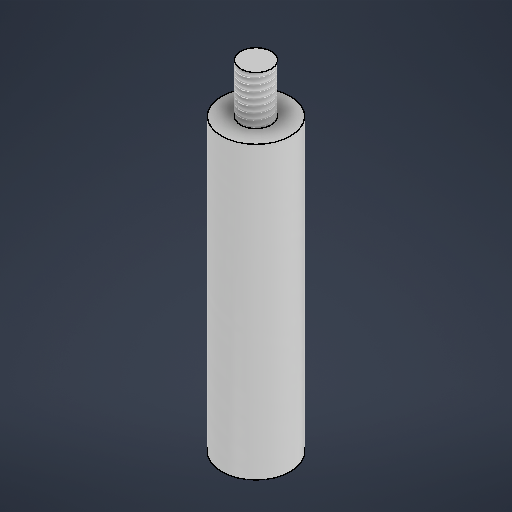
# Autodesk Inventor part: Joint Spacer
Saved by Autodesk Inventor 2026 (Build 300175050, 175E)
## iProperties
Created: 2025-05-26
Part Number: Joint Spacer
Material: Aluminum 6061
Document SubType Name: Modeling
Designer: Joshua Eah
Density: 2.7 g/cm^3
Appearance: Aluminum - Flat
Author: Joshua Eah
Autodesk Inventor part; units mm, degrees
ref_plane "YZ Plane" through (0, 0, 0) normal (1, 0, 0) x (0, 1, 0)
ref_plane "XZ Plane" through (0, 0, 0) normal (0, 1, 0) x (-1, 0, 0)
ref_plane "XY Plane" through (0, 0, 0) normal (0, 0, 1) x (1, 0, 0)
sketch "Sketch1" plane through (0, 0, 0) normal (0, 1, 0) x (-1, 0, 0)
  circle A0 centre (0, 0) radius 2.25
  dimension "d0" = 4.5
  constraints: 1 centre point, 1 coincident
  measures "d0" diameter of A0
extrude "Extrusion1" add sketch "Sketch1" along normal blind 19
hole "Hole1" at (0, 0, 0) direction (0, 1, 0) diameter 1.567 depth 12.7 tip angle 118 thread size "M2x0.4" class "6H" standard "ANSI Metric M Profile"
sketch "Sketch2" plane through (0, 19, 0) normal (0, 1, 0) x (1, 0, 0)
  circle A0 centre (0, 0) radius 1
  dimension "d13" = 2
  constraints: 1 centre point, 1 coincident
  measures "d13" diameter of A0
extrude "Extrusion3" add sketch "Sketch2" along normal blind 3.175
thread "Thread1" size "M2x0.4" class "6g" standard "ANSI Metric M Profile" full length
body "Solid1"
